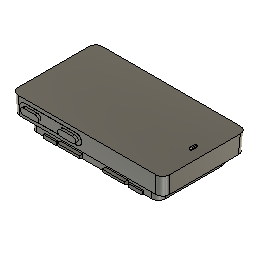
flat-surface-mount (Autodesk Fusion 360 archive; units mm, degrees)
design "esl module"
Autodesk Fusion 360 part; units mm, degrees
sketch "main-upper" plane through (0, 0, 0) normal (0, 0, 1) x (1, 0, 0)
  line L0 (33.55, 18.7) -> (-33.55, 18.7)
  line L1 (-33.55, 18.7) -> (-33.55, -18.7)
  line L2 (-33.55, -18.7) -> (33.55, -18.7)
  line L3 (33.55, -18.7) -> (33.55, 18.7)
  line L4 (33.55, 18.7) -> (-33.55, -18.7) construction
  line L5 (-33.55, 18.7) -> (33.55, -18.7) construction
  dimension "d1" = 67.1
  dimension "d2" = 37.4
  constraint horizontal L0
  constraint perpendicular L0 L1
  constraint parallel L0 L2
  constraint parallel L1 L3
  constraint coincident L4 origin
  constraint coincident L5 origin
  measures "d1" distance of L1.end L2.end
  measures "d2" distance of L0.end L1.end
extrude "Extrude1" add sketch "main-upper" against normal blind 8 draft -3
sketch "rgb-led" plane through (0, 0, 0) normal (0, 0, 1) x (-1, 0, 0)
  line L0 (-33.55, 18.7) -> (-33.55, -18.7)
  line L1 (-33.55, -18.7) -> (33.55, -18.7)
  line L2 (33.55, -18.7) -> (33.55, 18.7)
  line L3 (33.55, 18.7) -> (-33.55, 18.7)
  line L4 (-27.8, -1) -> (-27.8, 1)
  arc A0 (-27.8, 1) -> (-29.05, 1) centre (-28.425, 1) ccw
  line L5 (-29.05, 1) -> (-29.05, -1)
  arc A1 (-29.05, -1) -> (-27.8, -1) centre (-28.425, -1) ccw
  line L6 (-28.425, -1.625) -> (-28.425, 1.625) construction
  line L7 (-28.425, -18.7) -> (-28.425, 18.7) construction
  point P0 (-28.425, 0)
  point P1 (-28.425, 0)
  dimension "d5" = 3.25
  dimension "d6" = 1.25
  dimension "d8" = 4.5
  constraint tangent L4 A0
  constraint tangent A0 L5
  constraint parallel L4 L5
  constraint tangent L5 A1
  constraint tangent L4 A1
  constraint midpoint A1 L6.start
  constraint midpoint A0 L6.end
  constraint vertical L6
  constraint coincident L1 L7.start
  constraint coincident L3 L7.end
  constraint vertical L7
  constraint midpoint L7 P1
  constraint midpoint L6 P1
  constraint coincident P1 P0
  measures "d5" distance of L6.start L6.end
  measures "d6" distance of L4 L5
  measures "d8" distance of L0 L5
extrude "Extrude2" add sketch "rgb-led" along normal blind 0.6 contours L4 A0 L5 A1
fillet "Fillet1" radius 0.25 4 edges at (28.425, 1.625, 0.6) (27.8, 0, 0.6) (28.425, -1.625, 0.6) (29.05, 0, 0.6)
sketch "eink" plane through (0, 0, 0) normal (0, 0, 1) x (-1, 0, 0)
  line L0 (-29.05, -1) -> (-29.05, 1)
  arc A0 (-27.8, 1) -> (-29.05, 1) centre (-28.425, 1) ccw
  line L1 (-27.8, 1) -> (-27.8, -1)
  arc A1 (-29.05, -1) -> (-27.8, -1) centre (-28.425, -1) ccw
  line L2 (-33.55, 18.7) -> (-33.55, -18.7)
  line L3 (-33.55, -18.7) -> (33.55, -18.7)
  line L4 (33.55, -18.7) -> (33.55, 18.7)
  line L5 (33.55, 18.7) -> (-33.55, 18.7)
  line L6 (-24.05, 14) -> (24.05, 14)
  line L7 (24.05, 14) -> (24.05, -14)
  line L8 (24.05, -14) -> (-24.05, -14)
  line L9 (-24.05, -14) -> (-24.05, 14)
  line L10 (-24.05, 14) -> (24.05, -14) construction
  line L11 (24.05, 14) -> (-24.05, -14) construction
  dimension "d13" = 48.1
  dimension "d14" = 28
  constraint horizontal L6
  constraint perpendicular L6 L7
  constraint parallel L6 L8
  constraint parallel L7 L9
  constraint coincident L10 origin
  constraint coincident L11 origin
  measures "d13" distance of L7.end L8.end
  measures "d14" distance of L6.start L8.end
sketch "buttons-base" plane through (0, -18.6488, -0.9773) normal (0, -0.99863, -0.052336) x (1, 0, 0)
  line L0 (-33.1307, -7.0323) -> (33.1307, -7.0323)
  line L1 (33.1307, -7.0323) -> (33.55, 0.9787)
  line L2 (33.55, 0.9787) -> (-33.55, 0.9787)
  line L3 (-33.55, 0.9787) -> (-33.1307, -7.0323)
  line L4 (-27.65, -5.4713) -> (-4.95, -5.4713)
  arc A0 (-4.95, -5.4713) -> (-4.95, -0.6713) centre (-4.95, -3.0713) ccw
  line L5 (-4.95, -0.6713) -> (-27.65, -0.6713)
  arc A1 (-27.65, -0.6713) -> (-27.65, -5.4713) centre (-27.65, -3.0713) ccw
  line L6 (-30.05, -3.0713) -> (-2.55, -3.0713) construction
  dimension "d15" = 4.8
  dimension "d16" = 27.5
  dimension "d17" = 1.65
  dimension "d19" = 3.5
  constraint tangent L4 A0
  constraint tangent A0 L5
  constraint parallel L4 L5
  constraint tangent L5 A1
  constraint tangent L4 A1
  constraint midpoint A1 L6.start
  constraint midpoint A0 L6.end
  constraint parallel L0 L6
  measures "d15" distance of L4 L5
  measures "d16" distance of L6.start L6.end
  measures "d17" distance of L2 L5
  measures "d19" horizontal distance of L2.end L6.start
sketch "buttons" plane through (0, -18.6488, -0.9773) normal (0, -0.99863, -0.052336) x (1, 0, 0)
  line L0 (-27.15, -4.4713) -> (-21.95, -4.4713)
  arc A0 (-21.95, -4.4713) -> (-21.95, -1.6713) centre (-21.95, -3.0713) ccw
  line L1 (-21.95, -1.6713) -> (-27.15, -1.6713)
  arc A1 (-27.15, -1.6713) -> (-27.15, -4.4713) centre (-27.15, -3.0713) ccw
  line L2 (-28.55, -3.0713) -> (-20.55, -3.0713) construction
  line L3 (-30.05, -3.0713) -> (-2.55, -3.0713)
  line L4 (-27.65, -5.4713) -> (-4.95, -5.4713)
  line L5 (-16.3, -3.0713) -> (-16.3, -5.4713) construction
  line L6 (-5.45, -4.4713) -> (-10.65, -4.4713)
  arc A2 (-10.65, -1.6713) -> (-10.65, -4.4713) centre (-10.65, -3.0713) ccw
  line L7 (-10.65, -1.6713) -> (-5.45, -1.6713)
  arc A3 (-5.45, -4.4713) -> (-5.45, -1.6713) centre (-5.45, -3.0713) ccw
  dimension "d20" = 8
  dimension "d21" = 2.8
  dimension "d22" = 1.5
  constraint tangent L0 A0
  constraint tangent A0 L1
  constraint parallel L0 L1
  constraint tangent L1 A1
  constraint tangent L0 A1
  constraint midpoint A1 L2.start
  constraint midpoint A0 L2.end
  constraint horizontal L2
  constraint collinear L2 L3
  constraint midpoint L3 L5.start
  constraint midpoint L4 L5.end
  constraint symmetric L0.start L5 L6.start
  constraint symmetric L0.end L5 L6.end
  constraint symmetric A0.end L5 A2.start
  constraint symmetric L1.end L5 L7.end
  constraint symmetric A0 L5 A2
  constraint symmetric A1 L5 A3
  measures "d20" distance of L2.start L2.end
  measures "d21" diameter of A0
  measures "d22" distance of L2.start L3.start
extrude "Extrude3" add sketch "buttons-base" along normal blind 0.1 contours L4 A0 L5 A1
extrude "Extrude4" add sketch "buttons" along normal blind 1.2
sketch "batery-compartment-body" plane through (0, 0, -8) normal (0, 0, -1) x (1, 0, 0)
  line L0 (-33.1307, -18.2807) -> (33.1307, -18.2807)
  line L1 (33.1307, -18.2807) -> (33.1307, 18.2807)
  line L2 (33.1307, 18.2807) -> (-33.1307, 18.2807)
  line L3 (-33.1307, 18.2807) -> (-33.1307, -18.2807)
  line L4 (-28.75, -15.7) -> (28.75, -15.7)
  line L5 (28.75, -15.7) -> (28.75, 15.7)
  line L6 (28.75, 15.7) -> (-28.75, 15.7)
  line L7 (-28.75, 15.7) -> (-28.75, -15.7)
  line L8 (-28.75, -15.7) -> (28.75, 15.7) construction
  line L9 (28.75, -15.7) -> (-28.75, 15.7) construction
  dimension "d27" = 57.5
  dimension "d28" = 31.4
  constraint horizontal L4
  constraint perpendicular L4 L5
  constraint parallel L4 L6
  constraint parallel L5 L7
  constraint coincident L8 origin
  constraint coincident L9 origin
  measures "d27" distance of L5.end L6.end
  measures "d28" distance of L4.end L5.end
extrude "Extrude5" add sketch "batery-compartment-body" along normal blind 5.4 draft -3 contours L4 L5 L6 L7
sketch "rear-label-indent" plane through (0, 0, -13.4) normal (0, 0, -1) x (1, 0, 0)
  line L0 (28.467, 15.417) -> (-28.467, 15.417)
  line L1 (-28.467, 15.417) -> (-28.467, -15.417)
  line L2 (-28.467, -15.417) -> (28.467, -15.417)
  line L3 (28.467, -15.417) -> (28.467, 15.417)
  line L4 (15.5, 12.5) -> (-15.5, 12.5)
  line L5 (-17.5, 10.5) -> (-17.5, -10.5)
  line L6 (-15.5, -12.5) -> (15.5, -12.5)
  line L7 (17.5, -10.5) -> (17.5, 10.5)
  line L8 (17.5, 12.5) -> (-17.5, -12.5) construction
  line L9 (-17.5, 12.5) -> (17.5, -12.5) construction
  line L10 (17.5, -10.5) -> (15.5, -12.5)
  line L11 (17.5, -12.5) -> (17.5, -10.5) construction
  line L12 (15.5, -12.5) -> (17.5, -12.5) construction
  arc A0 (-17.5, -10.5) -> (-15.5, -12.5) centre (-15.5, -10.5) ccw
  arc A1 (-15.5, 12.5) -> (-17.5, 10.5) centre (-15.5, 10.5) ccw
  arc A2 (17.5, 10.5) -> (15.5, 12.5) centre (15.5, 10.5) ccw
  dimension "d34" = 35
  dimension "d35" = 25
  dimension "d36" = 45
  dimension "d37" = 33
  dimension "d38" = 2
  dimension "d39" = 2
  dimension "d40" = 2
  constraint horizontal L4
  constraint perpendicular L4 L5
  constraint parallel L4 L6
  constraint parallel L5 L7
  constraint coincident L8 origin
  constraint coincident L9 origin
  constraint parallel L5 L11
  constraint parallel L4 L12
  constraint coincident L8.end L6
  constraint coincident L8.end L5
  constraint tangent L6 A0
  constraint tangent L5 A0
  constraint coincident L9.start L4
  constraint coincident L9.start L5
  constraint tangent L4 A1
  constraint tangent L5 A1
  constraint coincident L8.start L7
  constraint coincident L8.start L4
  constraint tangent L7 A2
  constraint tangent L4 A2
  measures "d34" distance of L8.end L9.end
  measures "d35" distance of L9.start L8.end
  measures "d36" angle of L7 L10
  measures "d37" distance of L8.end L6.end
  measures "d38" radius of A0
  measures "d39" radius of A1
  measures "d40" radius of A2
extrude "Extrude6" cut sketch "rear-label-indent" against normal blind 0.1 contours L4 L5 L6 L7 L10 A0 A1 A2
ref_plane "WorkPlane1" through (-28.467, 0, 0) normal (1, 0, 0) x (0, 1, 0)
sketch "clips-profiile" plane through (-28.467, 0, 0) normal (1, 0, 0) x (0, 1, 0)
  line L0 (15.417, -13.4) -> (-15.417, -13.4)
  line L1 (-15.417, -13.4) -> (-15.7, -8)
  line L2 (-15.7, -8) -> (15.7, -8)
  line L3 (15.7, -8) -> (15.417, -13.4)
  line L4 (-15.5218, -11.4) -> (-17.017, -11.4)
  line L5 (-17.017, -11.4) -> (-17.017, -12.4)
  line L6 (-17.017, -12.4) -> (-15.417, -13.4)
  line L7 (15.5218, -11.4) -> (17.267, -11.4)
  line L8 (17.267, -11.4) -> (17.267, -12.4)
  line L9 (17.267, -12.4) -> (15.417, -13.4)
  dimension "d49" = 2
  dimension "d50" = 1.6
  dimension "d51" = 1.85
  dimension "d52" = 1
  dimension "d53" = 1
  constraint coincident L1 L4.start
  constraint horizontal L4
  constraint perpendicular L4 L5
  constraint coincident L0.end L1.start
  constraint coincident L3 L7.start
  constraint perpendicular L7 L8
  constraint coincident L0.start L3.end
  constraint collinear L4 L7
  measures "d49" distance of L0.end L4
  measures "d50" distance of L0.end L5
  measures "d51" distance of L8 L0.start
  measures "d52" distance of L4.end L5.end
  measures "d53" distance of L7.end L8.end
fillet "Fillet2" radius 3 4 edges at (-33.3404, 18.4904, -4) (33.3404, 18.4904, -4) (33.3404, -18.4904, -4) (-33.3404, -18.4904, -4)
fillet "Fillet3" radius 3 4 edges at (28.6085, 15.5585, -10.7) (28.6085, -15.5585, -10.7) (-28.6085, -15.5585, -10.7) (-28.6085, 15.5585, -10.7)
extrude "Extrude7" add sketch "clips-profiile" along normal blind 48 from surface at 5 contours L3 L7 L8 L9 | L1 L4 L5 L6
sketch "clips-cut" plane through (0, 0, -11.4) normal (0, 0, 1) x (-1, 0, 0)
  line L0 (23.467, -17.267) -> (23.467, -15.5218)
  line L1 (23.467, -15.5218) -> (-24.533, -15.5218)
  line L2 (-24.533, -15.5218) -> (-24.533, -17.267)
  line L3 (-24.533, -17.267) -> (23.467, -17.267)
  line L4 (23.467, 15.5218) -> (23.467, 17.017)
  line L5 (23.467, 17.017) -> (-24.533, 17.017)
  line L6 (-24.533, 17.017) -> (-24.533, 15.5218)
  line L7 (-24.533, 15.5218) -> (23.467, 15.5218)
  line L8 (21.95, 18.6612) -> (27.15, 18.6612)
  line L9 (27.15, 18.6612) -> (27.15, 19.7597)
  line L10 (27.15, 19.7597) -> (21.95, 19.7597)
  line L11 (21.95, 19.7597) -> (21.95, 18.6612)
  line L12 (5.45, 18.6612) -> (10.65, 18.6612)
  line L13 (10.65, 18.6612) -> (10.65, 19.7597)
  line L14 (10.65, 19.7597) -> (5.45, 19.7597)
  line L15 (5.45, 19.7597) -> (5.45, 18.6612)
  line L16 (0, 0) -> (0, 30) construction
  line L17 (5, 15.5218) -> (5, 17.017)
  line L18 (15, 15.5218) -> (15, 17.017)
  line L19 (-15, 15.5218) -> (-15, 17.017)
  line L20 (-5, 15.5218) -> (-5, 17.017)
  line L21 (-10, -17.267) -> (-10, -15.5218)
  line L22 (10, -17.267) -> (10, -15.5218)
  line L23 (-1.25, -17.267) -> (-1.25, -15.5218)
  line L24 (1.25, -17.267) -> (1.25, -15.5218)
  dimension "d61" = 10
  dimension "d62" = 5
  dimension "d63" = 10
  dimension "d64" = 1.25
  constraint coincident L16.start origin
  constraint perpendicular L5 L16
  constraint coincident L7 L17.start
  constraint coincident L5 L17.end
  constraint perpendicular L5 L17
  constraint coincident L7 L18.start
  constraint coincident L5 L18.end
  constraint perpendicular L5 L18
  constraint symmetric L16 L17.start L20.start
  constraint symmetric L16 L17.end L20.end
  constraint symmetric L16 L18.start L19.start
  constraint symmetric L16 L18.end L19.end
  constraint coincident L3 L21.start
  constraint coincident L1 L21.end
  constraint perpendicular L1 L21
  constraint symmetric L16 L21.start L22.start
  constraint symmetric L16 L21.end L22.end
  constraint coincident L3 L23.start
  constraint coincident L1 L23.end
  constraint perpendicular L1 L23
  constraint symmetric L16 L23.start L24.start
  constraint symmetric L16 L23.end L24.end
  measures "d61" distance of L17 L18
  measures "d62" distance of L16 L17
  measures "d63" distance of L16 L21
  measures "d64" distance of L16 L23
extrude "Extrude9" cut sketch "clips-cut" against normal blind 2 draft 3 contours L4 L5 L7 L18 | L5 L7 L17 L20 | L5 L6 L7 L19
extrude "Extrude10" cut sketch "clips-cut" against normal blind 2 draft 3 contours L0 L1 L3 L22 | L1 L3 L23 L24 | L1 L2 L3 L21
chamfer "Chamfer1" distance 1.5 angle 45 2 edges at (1.2762, 17.267, -11.9) (-1.2762, 17.267, -11.9)
sketch "battery-door-tabs" plane through (0, 0, -13.4) normal (0, 0, -1) x (1, 0, 0)
  arc A0 (17.5, 10.5) -> (15.5, 12.5) centre (15.5, 10.5) ccw
  line L0 (17.5, 10.5) -> (17.5, -10.5)
  line L1 (17.5, -10.5) -> (15.5, -12.5)
  line L2 (15.5, -12.5) -> (-15.5, -12.5)
  arc A1 (-17.5, -10.5) -> (-15.5, -12.5) centre (-15.5, -10.5) ccw
  line L3 (-17.5, -10.5) -> (-17.5, 10.5)
  arc A2 (-15.5, 12.5) -> (-17.5, 10.5) centre (-15.5, 10.5) ccw
  line L4 (-15.5, 12.5) -> (15.5, 12.5)
  ellipse E0 centre (-25.4629, -12.4129) end of major axis (-27.59, -14.54) minor radius 3 (-28.467, -12.4211) -> (-25.4711, -15.417) ccw
  line L5 (-25.4711, -15.417) -> (-9.8952, -15.417)
  line L6 (-9.8952, -15.417) -> (-1.3548, -15.417)
  line L7 (-1.3548, -15.417) -> (1.3548, -15.417)
  line L8 (1.3548, -15.417) -> (9.8952, -15.417)
  line L9 (9.8952, -15.417) -> (25.4711, -15.417)
  ellipse E1 centre (25.4629, -12.4129) end of major axis (27.59, -14.54) minor radius 3 (25.4711, -15.417) -> (28.467, -12.4211) ccw
  line L10 (28.467, -12.4211) -> (28.467, 12.4211)
  ellipse E2 centre (25.4629, 12.4129) end of major axis (27.59, 14.54) minor radius 3 (28.467, 12.4211) -> (25.4711, 15.417) ccw
  line L11 (25.4711, 15.417) -> (14.8952, 15.417)
  line L12 (14.8952, 15.417) -> (5.1048, 15.417)
  line L13 (5.1048, 15.417) -> (-5.1048, 15.417)
  line L14 (-5.1048, 15.417) -> (-14.8952, 15.417)
  line L15 (-14.8952, 15.417) -> (-25.4711, 15.417)
  ellipse E3 centre (-25.4629, 12.4129) end of major axis (-27.59, 14.54) minor radius 3 (-25.4711, 15.417) -> (-28.467, 12.4211) ccw
  line L16 (-28.467, 12.4211) -> (-28.467, -12.4211)
  line L17 (-5.1048, 15.417) -> (-5.0524, 17.017)
  line L18 (-5.0524, 17.017) -> (-14.9476, 17.017)
  line L19 (-14.9476, 17.017) -> (-14.8952, 15.417)
  line L20 (-14.8952, 15.417) -> (-5.1048, 15.417)
  line L21 (-15.8952, 15.417) -> (-21.8952, 15.417)
  line L22 (-21.8952, 15.417) -> (-21.8952, 16.217)
  line L23 (-21.8952, 16.217) -> (-15.8952, 16.217)
  line L24 (-15.8952, 16.217) -> (-15.8952, 15.417)
  line L25 (-15.8952, 15.417) -> (-21.8952, 16.217) construction
  line L26 (-21.8952, 15.417) -> (-15.8952, 16.217) construction
  line L27 (0, 0) -> (0, 15.417) construction
  line L28 (15.8952, 16.217) -> (15.8952, 15.417)
  line L29 (21.8952, 15.417) -> (21.8952, 16.217)
  line L30 (21.8952, 16.217) -> (15.8952, 16.217)
  point P0 (-18.8952, 15.817)
  dimension "d75" = 0.8
  dimension "d76" = 6
  dimension "d77" = 1
  constraint horizontal L21
  constraint perpendicular L21 L22
  constraint parallel L21 L23
  constraint parallel L22 L24
  constraint coincident L25 P0
  constraint coincident L26 P0
  constraint collinear L15 L21
  constraint coincident L27.start origin
  constraint midpoint L13 L27.end
  constraint symmetric L21.start L27 L28.end
  constraint symmetric L21.end L27 L29.start
  constraint symmetric L22.end L27 L29.end
  constraint symmetric L23.end L27 L28.start
  measures "d75" distance of L21.end L22.end
  measures "d76" distance of L22.end L23.end
  measures "d77" distance of L14.end L24
extrude "Extrude11" add sketch "battery-door-tabs" against normal blind 1.5 contours L15 L21 L22 L23 L24 | L11 L28 L29 L30
equation "d4 = -body_draft_angle"
equation "d30 = -body_draft_angle"
equation "d64 = ( 2.5 / 2 ) * 1 mm"
equation "d66 = body_draft_angle"
equation "d68 = body_draft_angle"
equation "d71 = corner_radius"
equation "d73 = corner_radius"
equation "corner_radius = 3.0 mm" comment "exxterior corners are rounded"
equation "body_draft_angle = 3 deg" comment "Draft angle"
equation "pogo_pad = 1.5 mm" comment "dimension of pogo pad square"
